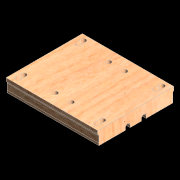
# Autodesk Inventor part: AXYZ
Saved by Autodesk Inventor 2016 (Build 200138000, 138)
## iProperties
Created: 2015-08-04
Part Number: AXYZ
Material: PC/ABS Plastic
Document SubType Name: Modeling
Designer: Jose
Density: 0.357273 g/cm^3
Appearance: Smooth - White
Mass: 110.75 g
Surface Area: 363.633 cm^2
Volume: 201.364 cm^3
Author: Jose
Autodesk Inventor part; units mm, degrees
ref_plane "YZ Plane" through (0, 0, 0) normal (1, 0, 0) x (0, 1, 0)
ref_plane "XZ Plane" through (0, 0, 0) normal (0, 1, 0) x (-1, 0, 0)
ref_plane "XY Plane" through (0, 0, 0) normal (0, 0, 1) x (1, 0, 0)
sketch "Sketch1" plane through (0, 0, 0) normal (0, 0, 1) x (1, 0, 0)
  circle A0 centre (10.5, 36.5) radius 3.05 projected
  circle A1 centre (-10.5, 36.5) radius 3.05 projected
  circle A2 centre (-10.5, -33.5) radius 3.05 projected
  circle A3 centre (10.5, -33.5) radius 3.05 projected
  line L0 (60, 51.5) -> (-60, 51.5) projected
  line L1 (-60, 51.5) -> (-60, -48.5) projected
  line L2 (-60, -48.5) -> (60, -48.5) projected
  line L3 (60, -48.5) -> (60, 51.5) projected
  circle A4 centre (51.5, 8.625) radius 3.05 projected
  circle A5 centre (-51.5, -5.625) radius 3.05 projected
  circle A6 centre (51.5, -5.625) radius 3.05 projected
  circle A7 centre (-51.5, 8.625) radius 3.05 projected
  arc A8 (-54.55, 36.5) -> (-48.45, 36.5) centre (-51.5, 36.5) ccw projected
  arc A9 (48.45, 36.5) -> (54.55, 36.5) centre (51.5, 36.5) ccw projected
  arc A10 (54.55, -33.5) -> (48.45, -33.5) centre (51.5, -33.5) ccw projected
  arc A11 (-48.45, -33.5) -> (-54.55, -33.5) centre (-51.5, -33.5) ccw projected
  arc A12 (-13.55, 8.625) -> (-7.45, 8.625) centre (-10.5, 8.625) ccw projected
  arc A13 (13.55, -5.625) -> (7.45, -5.625) centre (10.5, -5.625) ccw projected
  arc A14 (-7.45, -5.625) -> (-13.55, -5.625) centre (-10.5, -5.625) ccw projected
  arc A15 (7.45, 8.625) -> (13.55, 8.625) centre (10.5, 8.625) ccw projected
  line L4 (-48.45, -33.5) -> (-48.45, -41.5) projected
  arc A16 (-54.55, -41.5) -> (-48.45, -41.5) centre (-51.5, -41.5) ccw projected
  line L5 (-54.55, -41.5) -> (-54.55, -33.5) projected
  line L6 (54.55, -33.5) -> (54.55, -41.5) projected
  arc A17 (48.45, -41.5) -> (54.55, -41.5) centre (51.5, -41.5) ccw projected
  line L7 (48.45, -41.5) -> (48.45, -33.5) projected
  line L8 (-54.55, 36.5) -> (-54.55, 44.5) projected
  arc A18 (-48.45, 44.5) -> (-54.55, 44.5) centre (-51.5, 44.5) ccw projected
  line L9 (-48.45, 44.5) -> (-48.45, 36.5) projected
  line L10 (-7.45, -5.625) -> (-7.45, -13.625) projected
  arc A19 (-13.55, -13.625) -> (-7.45, -13.625) centre (-10.5, -13.625) ccw projected
  line L11 (-13.55, -13.625) -> (-13.55, -5.625) projected
  line L12 (13.55, -5.625) -> (13.55, -13.625) projected
  arc A20 (7.45, -13.625) -> (13.55, -13.625) centre (10.5, -13.625) ccw projected
  line L13 (7.45, -13.625) -> (7.45, -5.625) projected
  line L14 (13.55, 16.625) -> (13.55, 8.625) projected
  line L15 (7.45, 8.625) -> (7.45, 16.625) projected
  arc A21 (13.55, 16.625) -> (7.45, 16.625) centre (10.5, 16.625) ccw projected
  line L16 (54.55, 44.5) -> (54.55, 36.5) projected
  line L17 (48.45, 36.5) -> (48.45, 44.5) projected
  arc A22 (54.55, 44.5) -> (48.45, 44.5) centre (51.5, 44.5) ccw projected
  line L18 (-7.45, 16.625) -> (-7.45, 8.625) projected
  line L19 (-13.55, 8.625) -> (-13.55, 16.625) projected
  arc A23 (-7.45, 16.625) -> (-13.55, 16.625) centre (-10.5, 16.625) ccw projected
  point P0 (0, 0)
  point P1 (-51.375, 35)
  point P2 (51.375, 35)
  point P3 (51.375, -35)
  point P4 (-51.375, -35)
  point P5 (-10.5, 7.125)
  point P6 (10.5, -7.125)
  point P7 (-10.5, -7.125)
  point P8 (10.5, 7.125)
extrude "Extrusion1" add sketch "Sketch1" along normal blind 18 contours L3 L2 L1 L0 | A4 | A5 | A6 | A7 | L19 A23 L18 A12 | L12 A20 L13 A13 | L10 A19 L11 A14 | L15 A21 L14 A15
sketch "Sketch2" plane through (60, -48.5, 0) normal (1, 0, 0) x (0, 0, -1)
  arc A0 (-3.1, 63.55) -> (-3.1, 57.45) centre (-3.1, 60.5) ccw
  arc A1 (-3.1, 42.55) -> (-3.1, 36.45) centre (-3.1, 39.5) ccw
  line L0 (0, 0) -> (0, 100) projected
  line L1 (0, 100) -> (-18, 100) projected
  line L2 (-18, 0) -> (-18, 100) projected
  line L3 (0, 0) -> (-18, 0) projected
  circle A2 centre (66.9, 39.625) radius 3.05 construction
  circle A3 centre (66.9, 60.375) radius 3.05 construction
  circle A4 centre (-3.1, 60.375) radius 3.05 construction
  circle A5 centre (-3.1, 39.625) radius 3.05 construction
  line L4 (81.9, -10) -> (81.9, 110) construction
  line L5 (81.9, 110) -> (-18.1, 110) construction
  line L6 (-18.1, 110) -> (-18.1, -10) construction
  line L7 (-18.1, -10) -> (81.9, -10) construction
  line L8 (-3.1, -4.425) -> (0, -4.425)
  line L9 (0, -4.425) -> (0, 1.675)
  line L10 (0, 1.675) -> (-3.1, 1.675)
  line L11 (0, 100) -> (0, 0) projected
  line L12 (-3.1, 36.45) -> (0, 36.45)
  line L13 (0, 36.45) -> (0, 42.55)
  line L14 (0, 42.55) -> (-3.1, 42.55)
  line L15 (-3.1, 57.45) -> (0, 57.45)
  line L16 (0, 57.45) -> (0, 63.55)
  line L17 (0, 63.55) -> (-3.1, 63.55)
  line L18 (-3.1, 98.325) -> (0, 98.325)
  line L19 (0, 98.325) -> (0, 104.425)
  line L20 (0, 104.425) -> (-3.1, 104.425)
  line L21 (-3.1, -1.375) -> (-3.1, 101.375) construction
  line L22 (-3.1, 60.5) -> (-3.1, 39.5) construction
  circle A6 centre (39.025, -1.875) radius 3.05 projected
  circle A7 centre (24.775, 101.875) radius 3.05 projected
  circle A8 centre (24.775, -1.875) radius 3.05 projected
  circle A9 centre (39.025, 101.875) radius 3.05 projected
  arc A10 (66.9, 104.925) -> (66.9, 98.825) centre (66.9, 101.875) ccw projected
  arc A11 (66.9, 1.175) -> (66.9, -4.925) centre (66.9, -1.875) ccw projected
  arc A12 (-3.1, -4.925) -> (-3.1, 1.175) centre (-3.1, -1.875) ccw projected
  arc A13 (-3.1, 98.825) -> (-3.1, 104.925) centre (-3.1, 101.875) ccw projected
  arc A14 (39.025, 63.425) -> (39.025, 57.325) centre (39.025, 60.375) ccw projected
  arc A15 (24.775, 36.575) -> (24.775, 42.675) centre (24.775, 39.625) ccw projected
  arc A16 (24.775, 57.325) -> (24.775, 63.425) centre (24.775, 60.375) ccw projected
  arc A17 (39.025, 42.675) -> (39.025, 36.575) centre (39.025, 39.625) ccw projected
  line L23 (-3.1, 98.825) -> (-11.1, 98.825) projected
  arc A18 (-11.1, 104.925) -> (-11.1, 98.825) centre (-11.1, 101.875) ccw projected
  line L24 (-11.1, 104.925) -> (-3.1, 104.925) projected
  line L25 (-3.1, -4.925) -> (-11.1, -4.925) projected
  arc A19 (-11.1, 1.175) -> (-11.1, -4.925) centre (-11.1, -1.875) ccw projected
  line L26 (-11.1, 1.175) -> (-3.1, 1.175) projected
  line L27 (66.9, 104.925) -> (74.9, 104.925) projected
  arc A20 (74.9, 98.825) -> (74.9, 104.925) centre (74.9, 101.875) ccw projected
  line L28 (74.9, 98.825) -> (66.9, 98.825) projected
  line L29 (24.775, 57.325) -> (16.775, 57.325) projected
  arc A21 (16.775, 63.425) -> (16.775, 57.325) centre (16.775, 60.375) ccw projected
  line L30 (16.775, 63.425) -> (24.775, 63.425) projected
  line L31 (24.775, 36.575) -> (16.775, 36.575) projected
  arc A22 (16.775, 42.675) -> (16.775, 36.575) centre (16.775, 39.625) ccw projected
  line L32 (16.775, 42.675) -> (24.775, 42.675) projected
  line L33 (47.025, 36.575) -> (39.025, 36.575) projected
  line L34 (39.025, 42.675) -> (47.025, 42.675) projected
  arc A23 (47.025, 36.575) -> (47.025, 42.675) centre (47.025, 39.625) ccw projected
  line L35 (74.9, -4.925) -> (66.9, -4.925) projected
  line L36 (66.9, 1.175) -> (74.9, 1.175) projected
  arc A24 (74.9, -4.925) -> (74.9, 1.175) centre (74.9, -1.875) ccw projected
  line L37 (47.025, 57.325) -> (39.025, 57.325) projected
  line L38 (39.025, 63.425) -> (47.025, 63.425) projected
  arc A25 (47.025, 57.325) -> (47.025, 63.425) centre (47.025, 60.375) ccw projected
  point P0 (0, 48.5)
  point P1 (-3.1, 50)
  point P2 (-18, 50)
  point P3 (-3.1, 50)
  point P4 (-3.1, 50)
  point P5 (-3.1, 50)
  point P6 (-3.1, 50)
  point P7 (66.9, 101.375)
  point P8 (66.9, -1.375)
  point P9 (-3.1, -1.375)
  point P10 (-3.1, 101.375)
  point P11 (39.025, 60.5)
  point P12 (24.775, 39.5)
  point P13 (24.775, 60.5)
  point P14 (39.025, 39.5)
  dimension "d2" = 6.1
  dimension "d3" = 3.1
  dimension "d4" = 21
  dimension "d5" = 102.75
  dimension "d6" = 6.1
  dimension "d7" = 6.1
  dimension "d8" = 6.1
  constraints: 28 end point, 4 coincident, 4 horizontal, 4 parallel, 4 perpendicular, 4 point on circle, 4 point on line, 3 midpoint, 3 vertical alignment, 2 centre point, 1 collinear, 1 equal radius, 1 horizontal alignment, 1 vertical, 10 other
  measures "d3" distance from line of L0 L22.end
  measures "d4" distance of L22.end L22.start
  measures "d5" distance of L21.start L21.end
  measures "d6" distance between parallel lines of L15 L17
  measures "d7" distance between parallel lines of L18 L20
  measures "d8" distance between parallel lines of L8 L10
sketch "Sketch2 outline for Extrusion2" plane through (60, -48.5, 0) normal (1, 0, 0) x (0, 0, -1)
  line L0 (-11.1, -4.925) -> (-3.1, -4.925)
  arc A0 (-11.1, 1.175) -> (-11.1, -4.925) centre (-11.1, -1.875) ccw
  line L1 (-3.1, 1.175) -> (-11.1, 1.175)
  line L2 (0, 1.675) -> (-3.1, 1.175)
  line L3 (0, -4.425) -> (0, 1.675)
  line L4 (-3.1, -4.925) -> (0, -4.425)
  line L5 (0, 104.425) -> (0, 98.325)
  line L6 (0, 98.325) -> (-3.1, 98.825)
  line L7 (-3.1, 98.825) -> (-11.1, 98.825)
  arc A1 (-11.1, 98.825) -> (-11.1, 104.925) centre (-11.1, 101.875) cw
  line L8 (-11.1, 104.925) -> (-3.1, 104.925)
  line L9 (-3.1, 104.925) -> (0, 104.425)
  line L10 (0, 36.45) -> (0, 42.55)
  line L11 (-3.1, 36.45) -> (0, 36.45)
  arc A2 (-3.1, 42.55) -> (-3.1, 36.45) centre (-3.1, 39.5) ccw
  line L12 (0, 42.55) -> (-3.1, 42.55)
  line L13 (0, 57.45) -> (0, 63.55)
  line L14 (-3.1, 57.45) -> (0, 57.45)
  arc A3 (-3.1, 63.55) -> (-3.1, 57.45) centre (-3.1, 60.5) ccw
  line L15 (0, 63.55) -> (-3.1, 63.55)
extrude "Extrusion2" cut sketch "Sketch2 outline for Extrusion2" against normal through all
body "Solid1"
